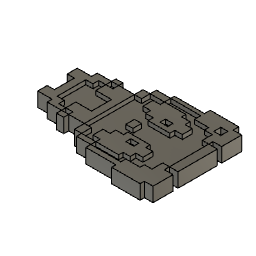
panda-keychain (Autodesk Fusion 360 design; units mm, degrees)
Autodesk Fusion 360 part; units mm, degrees
note: some values were not read from the file. Chosen so that the rebuilt part matches the saved one: which bodies a step acts on.
sketch "Sketch1" plane through (0, 0, 0) normal (0, 0, 1) x (1, 0, 0)
  line L0 (-15.7131, -43.8712) -> (-30, -43.8712)
  line L1 (-30, -43.8712) -> (-30, -50)
  line L2 (-30, -50) -> (-15.7131, -50)
  line L3 (-15.7131, -50) -> (-15.7131, -43.8712)
  line L4 (0, 49) -> (9, 49)
  line L5 (9, 49) -> (9, 53)
  line L6 (9, 53) -> (19, 53)
  line L7 (19, 53) -> (19, 56)
  line L8 (19, 56) -> (24, 56)
  line L9 (24, 56) -> (24, 53)
  line L10 (24, 53) -> (35, 53)
  line L11 (35, 53) -> (35, 59)
  line L12 (35, 59) -> (40, 59)
  line L13 (40, 59) -> (40, 63.4077)
  line L14 (40, 63.4077) -> (50, 63.4077)
  line L15 (50, 63.4077) -> (50, 66)
  line L16 (50, 66) -> (71, 66)
  line L17 (71, 66) -> (71, 70)
  line L18 (71, 70) -> (91, 70)
  line L19 (91, 70) -> (91, 66)
  line L20 (91, 66) -> (97, 66)
  line L21 (97, 66) -> (97, 52)
  line L22 (97, 52) -> (91, 52)
  line L23 (91, 52) -> (91, 49)
  line L24 (91, 49) -> (97, 49)
  line L25 (45, 49) -> (45, 56)
  line L26 (45, 56) -> (50, 56)
  line L27 (50, 56) -> (50, 59)
  line L28 (50, 59) -> (65, 59)
  line L29 (65, 59) -> (65, 56)
  line L30 (65, 56) -> (71, 56)
  line L31 (71, 56) -> (71, 52.5)
  line L32 (71, 52.5) -> (76, 52.5)
  line L33 (76, 52.5) -> (76, 45.5)
  line L34 (76, 45.5) -> (70.7717, 45.5)
  line L35 (60.6732, 48.9739) -> (66, 48.9739)
  line L36 (66, 48.9739) -> (66, 45.29)
  line L37 (66, 45.29) -> (60.6732, 45.29)
  line L38 (60.6732, 45.29) -> (60.6732, 48.9739)
  line L39 (45, 49) -> (50.3102, 49)
  line L40 (50.3102, 49) -> (50.3102, 45.531)
  line L41 (50.3102, 45.531) -> (55.5778, 45.531)
  line L42 (55.5778, 45.531) -> (55.5778, 42)
  line L43 (55.5778, 42) -> (70.7717, 42)
  line L44 (70.7717, 42) -> (70.7717, 45.5)
  line L45 (50, 38) -> (55, 38)
  line L46 (55, 38) -> (55, 32)
  line L47 (55, 32) -> (50, 32)
  line L48 (50, 32) -> (50, 38)
  line L49 (71, 25) -> (76, 25)
  line L50 (76, 25) -> (76, 18)
  line L51 (76, 18) -> (71, 18)
  line L52 (71, 18) -> (71, 14)
  line L53 (71, 14) -> (66, 14)
  line L54 (66, 14) -> (66, 11)
  line L55 (66, 11) -> (50, 11)
  line L56 (50, 11) -> (50, 14)
  line L57 (50, 14) -> (45, 14)
  line L58 (45, 14) -> (45, 21)
  line L59 (45, 21) -> (50, 21)
  line L60 (50, 21) -> (50, 25)
  line L61 (50, 25) -> (55.446, 25)
  line L62 (55.446, 25) -> (55.446, 28)
  line L63 (55.446, 28) -> (71, 28)
  line L64 (71, 28) -> (71, 25)
  line L65 (60.5, 25) -> (60.5, 21.5)
  line L66 (60.5, 21.5) -> (66, 21.5)
  line L67 (66, 21.5) -> (66, 25)
  line L68 (66, 25) -> (60.5, 25)
  line L69 (97, 49) -> (97, 21.5)
  line L70 (97, 21.5) -> (91, 21.5)
  line L71 (91, 21.5) -> (91, 18)
  line L72 (91, 18) -> (97, 18)
  line L73 (97, 18) -> (97, 4)
  line L74 (97, 4) -> (91, 4)
  line L75 (91, 4) -> (91, 1)
  line L76 (91, 1) -> (71, 1)
  line L77 (71, 1) -> (71, 4)
  line L78 (71, 4) -> (50, 4)
  line L79 (50, 4) -> (50, 7.5055)
  line L80 (50, 7.5055) -> (40, 7.5055)
  line L81 (40, 7.5055) -> (40, 11)
  line L82 (40, 11) -> (35, 11)
  line L83 (35, 11) -> (35, 18)
  line L84 (35, 18) -> (24, 18)
  line L85 (24, 18) -> (24, 14.5)
  line L86 (24, 14.5) -> (19, 14.5)
  line L87 (19, 14.5) -> (19, 18)
  line L88 (19, 18) -> (9, 18)
  line L89 (9, 18) -> (9, 21.4049)
  line L90 (9, 21.4049) -> (-1, 21.4049)
  line L91 (-1, 21.4049) -> (-1, 28)
  line L92 (-1, 28) -> (4, 28)
  line L93 (4, 28) -> (4, 42)
  line L94 (4, 42) -> (-1, 42)
  line L95 (-1, 42) -> (-1, 49)
  line L96 (-1, 49) -> (0, 49)
  line L97 (9, 25) -> (9, 45)
  line L98 (9, 45) -> (14, 45)
  line L99 (14, 45) -> (14, 49)
  line L100 (14, 49) -> (19, 49)
  line L101 (19, 49) -> (19, 53)
  line L102 (19, 53) -> (24, 53)
  line L103 (24, 49) -> (19, 49)
  line L104 (24, 49) -> (24, 53)
  line L105 (19, 49) -> (19, 42)
  line L106 (19, 42) -> (30, 42)
  line L107 (30, 42) -> (30, 28)
  line L108 (30, 28) -> (19, 28)
  line L109 (19, 28) -> (19, 21)
  line L110 (19, 21) -> (24, 21)
  line L111 (24, 21) -> (24, 18)
  line L112 (19, 18) -> (24, 18)
  line L113 (19, 18) -> (19, 21)
  line L114 (19, 21) -> (14, 21)
  line L115 (14, 21) -> (14, 25)
  line L116 (14, 25) -> (9, 25)
  line L117 (35, 53) -> (35, 18)
  line L118 (40, 18) -> (40, 11)
  line L119 (40, 18) -> (35, 18)
  line L120 (35, 53) -> (40, 53)
  line L121 (40, 53) -> (40, 59)
  line L122 (50, 59) -> (40, 59)
  line L123 (50, 63.4077) -> (50, 59)
  line L124 (50, 63.4077) -> (71, 63.4077)
  line L125 (71, 63.4077) -> (71, 59)
  line L126 (71, 59) -> (81, 59)
  line L127 (81, 59) -> (81, 56)
  line L128 (81, 56) -> (86.4762, 56)
  line L129 (86.4762, 56) -> (86.4762, 49)
  line L130 (86.4762, 49) -> (91, 49)
  line L131 (91, 49) -> (91, 21.5)
  line L132 (86.2751, 21.5) -> (86.2751, 14)
  line L133 (86.2751, 14) -> (81, 14)
  line L134 (81, 14) -> (81, 11)
  line L135 (81, 11) -> (71, 11)
  line L136 (71, 11) -> (71, 7.5055)
  line L137 (71, 7.5055) -> (50, 7.5055)
  line L138 (50, 7.5055) -> (50, 11)
  line L139 (40, 11) -> (50, 11)
  line L140 (86.2751, 21.5) -> (91, 21.5)
  line L141 (85.0529, 63.4077) -> (85.0529, 58.4606)
  line L142 (85.0529, 58.4606) -> (90, 58.4606)
  line L143 (90, 58.4606) -> (90, 63.4077)
  line L144 (90, 63.4077) -> (85.0529, 63.4077)
  constraint horizontal L0
  constraint vertical L1
  constraint horizontal L2
  constraint vertical L3
  constraint horizontal L4
  constraint perpendicular L4 L5
  constraint perpendicular L5 L6
  constraint perpendicular L6 L7
  constraint perpendicular L7 L8
  constraint perpendicular L8 L9
  constraint perpendicular L9 L10
  constraint perpendicular L10 L11
  constraint perpendicular L11 L12
  constraint perpendicular L12 L13
  constraint perpendicular L13 L14
  constraint perpendicular L14 L15
  constraint perpendicular L15 L16
  constraint perpendicular L16 L17
  constraint perpendicular L17 L18
  constraint perpendicular L18 L19
  constraint perpendicular L19 L20
  constraint perpendicular L20 L21
  constraint perpendicular L21 L22
  constraint perpendicular L22 L23
  constraint perpendicular L21 L24
  constraint vertical L25
  constraint perpendicular L25 L26
  constraint perpendicular L26 L27
  constraint perpendicular L27 L28
  constraint perpendicular L28 L29
  constraint perpendicular L29 L30
  constraint perpendicular L30 L31
  constraint perpendicular L31 L32
  constraint perpendicular L32 L33
  constraint perpendicular L33 L34
  constraint parallel L28 L35
  constraint perpendicular L35 L36
  constraint perpendicular L36 L37
  constraint perpendicular L35 L38
  constraint perpendicular L25 L39
  constraint perpendicular L39 L40
  constraint perpendicular L40 L41
  constraint perpendicular L39 L42
  constraint perpendicular L42 L43
  constraint perpendicular L43 L44
  constraint horizontal L45
  constraint perpendicular L45 L46
  constraint perpendicular L46 L47
  constraint horizontal L49
  constraint perpendicular L49 L50
  constraint perpendicular L50 L51
  constraint perpendicular L51 L52
  constraint perpendicular L52 L53
  constraint perpendicular L53 L54
  constraint perpendicular L54 L55
  constraint perpendicular L55 L56
  constraint perpendicular L56 L57
  constraint perpendicular L55 L58
  constraint perpendicular L58 L59
  constraint perpendicular L59 L60
  constraint perpendicular L60 L61
  constraint perpendicular L61 L62
  constraint perpendicular L60 L63
  constraint perpendicular L49 L64
  constraint perpendicular L49 L65
  constraint perpendicular L65 L66
  constraint perpendicular L49 L67
  constraint perpendicular L24 L69
  constraint perpendicular L69 L70
  constraint perpendicular L70 L71
  constraint perpendicular L71 L72
  constraint perpendicular L72 L73
  constraint perpendicular L73 L74
  constraint perpendicular L74 L75
  constraint perpendicular L75 L76
  constraint perpendicular L76 L77
  constraint perpendicular L77 L78
  constraint perpendicular L78 L79
  constraint perpendicular L79 L80
  constraint perpendicular L78 L81
  constraint perpendicular L81 L82
  constraint perpendicular L82 L83
  constraint perpendicular L81 L84
  constraint perpendicular L84 L85
  constraint perpendicular L85 L86
  constraint perpendicular L84 L87
  constraint perpendicular L87 L88
  constraint perpendicular L86 L89
  constraint perpendicular L87 L90
  constraint perpendicular L90 L91
  constraint perpendicular L87 L92
  constraint perpendicular L92 L93
  constraint perpendicular L93 L94
  constraint perpendicular L92 L95
  constraint perpendicular L95 L96
  constraint vertical L97
  constraint perpendicular L97 L98
  constraint perpendicular L98 L99
  constraint perpendicular L99 L100
  constraint perpendicular L100 L101
  constraint perpendicular L9 L102
  constraint perpendicular L101 L103
  constraint perpendicular L10 L104
  constraint perpendicular L100 L105
  constraint perpendicular L101 L106
  constraint perpendicular L106 L107
  constraint perpendicular L107 L108
  constraint perpendicular L108 L109
  constraint perpendicular L109 L110
  constraint perpendicular L85 L112
  constraint perpendicular L110 L113
  constraint perpendicular L110 L111
  constraint perpendicular L113 L114
  constraint perpendicular L114 L115
  constraint perpendicular L97 L116
  constraint perpendicular L84 L117
  constraint perpendicular L82 L118
  constraint perpendicular L83 L119
  constraint perpendicular L117 L120
  constraint perpendicular L27 L122
  constraint perpendicular L122 L123
  constraint perpendicular L123 L124
  constraint perpendicular L32 L125
  constraint perpendicular L125 L126
  constraint perpendicular L32 L127
  constraint perpendicular L127 L128
  constraint perpendicular L32 L129
  constraint perpendicular L23 L130
  constraint perpendicular L70 L131
  constraint perpendicular L70 L132
  constraint perpendicular L132 L133
  constraint perpendicular L133 L134
  constraint perpendicular L134 L135
  constraint perpendicular L133 L136
  constraint perpendicular L136 L137
  constraint perpendicular L55 L138
  constraint perpendicular L138 L139
  constraint perpendicular L71 L140
  constraint perpendicular L124 L141
  constraint perpendicular L141 L142
  constraint perpendicular L124 L143
  constraint perpendicular L141 L144
  constraint equal L143 L144
extrude "Extrude1" add sketch "Sketch1" along normal blind 10 contours L4 L5 L6 L88 L89 L90 L91 L92 L93 L94 L95 L96 L97 L98 L99 L100 L101 L113 L114 L115 L116 | L7 L8 L9 L102 | L10 L84 L103 L104 L105 L106 L107 L108 L109 L110 L111 L117 | L49 L50 L51 L52 L53 L54 L55 L56 L57 L58 L59 L60 L61 L62 L63 L64 | L25 L26 L27 L28 L29 L30 L31 L32 L33 L34 L39 L40 L41 L42 L43 L44 | L11 L12 L120 L121 | L82 L83 L118 L119 | L13 L14 L122 L123 | L85 L86 L87 L112 | L80 L81 L138 L139 | L15 L16 L17 L18 L19 L20 L21 L22 L23 L124 L125 L126 L127 L128 L129 L130 | L71 L72 L73 L74 L75 L76 L77 L78 L79 L132 L133 L134 L135 L136 L137 L140 | L24 L69 L70 L131 | L45 L46 L47 L48 makes body 1 at (82.351, 67.8026, 0) makes body 1 at (43.3333, 63.4077, 3.3333) makes body 1 at (58.5577, 53.658, 0) makes body 1 at (40, 55, 3.3333) makes body 1 at (91, 39.8333, 3.3333) makes body 1 at (81, 4.3333, 0) makes body 1 at (29.6667, 48, 0) makes body 1 at (20.6667, 56, 3.3333) makes body 1 at (40, 15.6667, 3.3333) makes body 1 at (4, 46.6667, 0) makes body 1 at (20.6667, 18, 3.3333) makes body 1 at (46.6667, 7.5055, 3.3333) makes body 1 at (58.8333, 16.5, 0) makes body 2 at (50, 34, 3.3333)
sketch "Sketch2" plane through (0, 0, 0) normal (0, 0, 1) x (1, 0, 0)
  line L0 (19, 53) -> (24, 53)
  line L1 (24, 53) -> (24, 49)
  line L2 (24, 49) -> (19, 49)
  line L3 (19, 49) -> (19, 53)
  line L4 (14, 45) -> (14, 49)
  line L5 (14, 49) -> (19, 49)
  line L6 (19, 42) -> (30, 42)
  line L7 (30, 42) -> (30, 28)
  line L8 (30, 28) -> (19, 28)
  line L9 (19, 28) -> (19, 21)
  line L10 (19, 21) -> (14, 21)
  line L11 (14, 21) -> (14, 25)
  line L12 (14, 25) -> (9, 25)
  line L13 (9, 25) -> (9, 45)
  line L14 (9, 45) -> (14, 45)
  line L15 (19, 49) -> (19, 42)
  line L16 (19, 21) -> (24, 21)
  line L17 (24, 21) -> (24, 18)
  line L18 (24, 18) -> (19, 18)
  line L19 (19, 18) -> (19, 21)
  line L20 (66, 49) -> (60.5621, 49)
  line L21 (60.5621, 49) -> (60.5621, 45.2572)
  line L22 (60.5621, 45.2572) -> (66, 45.2572)
  line L23 (66, 45.2572) -> (66, 49)
  line L24 (66, 25) -> (60.5077, 25)
  line L25 (60.5077, 25) -> (60.5077, 21.5326)
  line L26 (60.5077, 21.5326) -> (66, 21.5326)
  line L27 (66, 21.5326) -> (66, 25)
  line L28 (50, 38) -> (55, 38)
  line L29 (55, 38) -> (55, 32)
  line L30 (55, 32) -> (50, 32)
  line L31 (50, 32) -> (50, 38)
  line L32 (70.8464, 45.4749) -> (70.8464, 42)
  line L33 (70.8464, 45.4749) -> (76, 45.4749)
  line L34 (76, 45.4749) -> (76, 52.4943)
  line L35 (76, 52.4943) -> (71, 52.4943)
  line L36 (71, 52.4943) -> (71, 56)
  line L37 (71, 56) -> (65, 56)
  line L38 (65, 56) -> (65, 59)
  line L39 (65, 59) -> (50, 59)
  line L40 (50, 59) -> (50, 63.5)
  line L41 (50, 63.5) -> (71, 63.5)
  line L42 (71, 63.5) -> (71, 59)
  line L43 (71, 59) -> (81, 59)
  line L44 (81, 59) -> (81, 56)
  line L45 (81, 56) -> (86.4364, 56)
  line L46 (86.4364, 56) -> (86.4364, 49)
  line L47 (86.4364, 49) -> (91, 49)
  line L48 (91, 49) -> (91, 21.5)
  line L49 (91, 21.5) -> (86.2722, 21.5)
  line L50 (86.2722, 21.5) -> (86.2722, 14)
  line L51 (86.2722, 14) -> (81, 14)
  line L52 (81, 14) -> (81, 11)
  line L53 (81, 11) -> (71, 11)
  line L54 (71, 11) -> (71, 7.5252)
  line L55 (71, 7.5252) -> (50, 7.5252)
  line L56 (50, 7.5252) -> (50, 11)
  line L57 (50, 11) -> (66, 11)
  line L58 (66, 11) -> (66, 14)
  line L59 (66, 14) -> (71, 14)
  line L60 (71, 14) -> (71, 18)
  line L61 (71, 18) -> (76, 18)
  line L62 (76, 18) -> (76, 25)
  line L63 (76, 25) -> (71, 25)
  line L64 (71, 25) -> (71, 28)
  line L65 (71, 28) -> (55.4589, 28)
  line L66 (55.4589, 28) -> (55.4589, 25)
  line L67 (55.4589, 25) -> (50, 25)
  line L68 (50, 25) -> (50, 21)
  line L69 (50, 21) -> (45, 21)
  line L70 (45, 21) -> (45, 14)
  line L71 (45, 14) -> (50, 14)
  line L72 (50, 14) -> (50, 11)
  line L73 (40, 11) -> (40, 18)
  line L74 (40, 18) -> (35, 18)
  line L75 (35, 18) -> (35, 53)
  line L76 (35, 53) -> (40, 53)
  line L77 (50, 56.0842) -> (45, 56.0842)
  line L78 (45, 56.0842) -> (45, 49)
  line L79 (45, 49) -> (50.3, 49)
  line L80 (50.3, 49) -> (50.3, 45.5)
  line L81 (50.3, 45.5) -> (55.5787, 45.5)
  line L82 (55.5787, 45.5) -> (55.5787, 42)
  line L83 (55.5787, 42) -> (70.8464, 42)
  line L84 (40, 11) -> (50, 11)
  line L85 (40, 53) -> (40, 59)
  line L86 (40, 59) -> (50, 59)
  line L87 (50, 56.0842) -> (50, 59)
  constraint horizontal L0
  constraint vertical L1
  constraint horizontal L2
  constraint vertical L3
  constraint vertical L4
  constraint perpendicular L4 L5
  constraint parallel L5 L6
  constraint perpendicular L6 L7
  constraint perpendicular L7 L8
  constraint perpendicular L8 L9
  constraint perpendicular L9 L10
  constraint perpendicular L10 L11
  constraint perpendicular L9 L12
  constraint perpendicular L12 L13
  constraint perpendicular L4 L14
  constraint perpendicular L6 L15
  constraint perpendicular L9 L16
  constraint perpendicular L16 L17
  constraint perpendicular L9 L18
  constraint perpendicular L10 L19
  constraint horizontal L20
  constraint vertical L21
  constraint horizontal L22
  constraint vertical L23
  constraint horizontal L24
  constraint vertical L25
  constraint horizontal L26
  constraint vertical L27
  constraint horizontal L28
  constraint vertical L29
  constraint horizontal L30
  constraint vertical L31
  constraint parallel L23 L32
  constraint perpendicular L32 L33
  constraint perpendicular L33 L34
  constraint perpendicular L34 L35
  constraint perpendicular L35 L36
  constraint perpendicular L34 L37
  constraint perpendicular L37 L38
  constraint perpendicular L38 L39
  constraint perpendicular L39 L40
  constraint perpendicular L40 L41
  constraint perpendicular L41 L42
  constraint perpendicular L42 L43
  constraint perpendicular L43 L44
  constraint perpendicular L42 L45
  constraint perpendicular L45 L46
  constraint perpendicular L46 L47
  constraint perpendicular L47 L48
  constraint perpendicular L48 L49
  constraint perpendicular L49 L50
  constraint perpendicular L50 L51
  constraint perpendicular L51 L52
  constraint perpendicular L50 L53
  constraint perpendicular L53 L54
  constraint perpendicular L54 L55
  constraint perpendicular L55 L56
  constraint perpendicular L56 L57
  constraint perpendicular L57 L58
  constraint perpendicular L58 L59
  constraint perpendicular L59 L60
  constraint perpendicular L60 L61
  constraint perpendicular L61 L62
  constraint perpendicular L62 L63
  constraint perpendicular L61 L64
  constraint perpendicular L64 L65
  constraint perpendicular L65 L66
  constraint perpendicular L66 L67
  constraint perpendicular L67 L68
  constraint perpendicular L68 L69
  constraint perpendicular L69 L70
  constraint perpendicular L68 L71
  constraint perpendicular L57 L72
  constraint perpendicular L57 L73
  constraint perpendicular L73 L74
  constraint perpendicular L74 L75
  constraint perpendicular L75 L76
  constraint perpendicular L40 L77
  constraint perpendicular L39 L78
  constraint perpendicular L78 L79
  constraint perpendicular L79 L80
  constraint perpendicular L80 L81
  constraint perpendicular L81 L82
  constraint perpendicular L32 L83
  constraint perpendicular L56 L84
  constraint perpendicular L76 L85
  constraint perpendicular L40 L86
  constraint perpendicular L86 L87
extrude "Extrude2" cut sketch "Sketch2" along normal blind 7 bodies 1
extrude "Extrude3" add sketch "Sketch2" along normal blind 7 bodies 1 2
named bodies: "panda"
